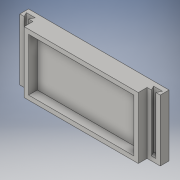
# Autodesk Inventor part: doveTailSide
Saved by Autodesk Inventor 2016 (Build 200138000, 138)
## iProperties
Created: 2015-11-04
Part Number: doveTailSide
Material: Generic
Document SubType Name: Modeling
Designer: rossmosier
Density: 1 g/cm^3
Appearance: Default
Author: rossmosier
Autodesk Inventor part; units mm, degrees
ref_plane "YZ Plane" through (0, 0, 0) normal (1, 0, 0) x (0, 1, 0)
ref_plane "XZ Plane" through (0, 0, 0) normal (0, 1, 0) x (-1, 0, 0)
ref_plane "XY Plane" through (0, 0, 0) normal (0, 0, 1) x (1, 0, 0)
sketch "Sketch2" plane through (0, 0, 0) normal (0, 0, 1) x (1, 0, 0)
  line L0 (0, 0) -> (203.2, 0)
  line L1 (203.2, 0) -> (203.2, 88.9)
  line L2 (203.2, 88.9) -> (0, 88.9)
  line L3 (0, 88.9) -> (0, 0)
  dimension "d6" = 203.2
  dimension "d7" = 88.9
  constraints: 8 end point, 2 parallel, 1 horizontal, 1 perpendicular
  measures "d6" distance of L2.end L1.end
  measures "d7" distance of L1.end L0.end
extrude "Extrusion2" add sketch "Sketch2" along normal blind 12.7
sketch "Sketch3" plane through (0, 0, 12.7) normal (0, 0, 1) x (1, 0, 0)
  line L0 (0, 0) -> (203.2, 0) projected
  line L1 (203.2, 0) -> (203.2, 88.9) projected
  line L2 (203.2, 88.9) -> (0, 88.9) projected
  line L3 (0, 88.9) -> (0, 0) projected
  line L4 (203.2, 88.9) -> (0, 88.9) construction
  line L5 (0, 0) -> (203.2, 0) construction
  line L6 (0, 88.9) -> (203.2, 0) construction
  line L7 (203.2, 0) -> (203.2, 88.9) construction
  line L8 (203.2, 88.9) -> (0, 0) construction
  line L9 (25.4, 6.35) -> (177.8, 6.35)
  line L10 (177.8, 6.35) -> (177.8, 82.55)
  line L11 (177.8, 82.55) -> (25.4, 82.55)
  line L12 (25.4, 82.55) -> (25.4, 6.35)
  line L13 (25.4, 6.35) -> (177.8, 82.55) construction
  line L14 (177.8, 6.35) -> (25.4, 82.55) construction
  line L15 (19.05, 88.9) -> (184.15, 88.9)
  line L16 (184.15, 88.9) -> (184.15, 0)
  line L17 (184.15, 0) -> (19.05, 0)
  line L18 (19.05, 0) -> (19.05, 88.9)
  point P0 (101.6, 44.45)
  dimension "d10" = 152.4
  dimension "d11" = 76.2
  dimension "d12" = 6.35
  constraints: 24 end point, 4 parallel, 3 midpoint, 2 perpendicular, 1 horizontal, 3 other
  measures "d10" distance of L11.end L10.end
  measures "d11" distance of L10.end L9.end
  measures "d12" distance between parallel lines of L11 L15
extrude "Extrusion3" add sketch "Sketch3" along normal blind 12.7 contours L18 L2 L16 L0
sketch "Sketch5" plane through (0, 88.9, 0) normal (0, 1, 0) x (1, 0, 0)
  line L0 (203.2, 0) -> (0, 0) projected
  line L1 (0, 0) -> (0, -12.7) projected
  line L2 (19.05, -12.7) -> (0, -12.7) projected
  line L3 (19.05, -12.7) -> (19.05, -25.4) projected
  line L4 (184.15, -25.4) -> (19.05, -25.4) projected
  line L5 (184.15, -12.7) -> (184.15, -25.4) projected
  line L6 (203.2, -12.7) -> (184.15, -12.7) projected
  line L7 (203.2, 0) -> (203.2, -12.7) projected
  line L8 (0, 0) -> (203.2, 0) construction
  line L9 (0, -12.7) -> (19.05, -12.7)
  line L10 (19.05, -12.7) -> (19.05, 0) construction
  line L11 (19.05, 0) -> (0, 0) construction
  line L12 (0, 0) -> (0, -12.7) construction
  line L13 (19.05, -12.7) -> (0, -12.7) construction
  line L14 (9.525, -12.7) -> (9.525, -6.3424) construction
  line L15 (9.525, -12.7) -> (12.7, -12.7) construction
  line L16 (9.525, -12.7) -> (6.35, -12.7)
  line L17 (9.525, -6.3424) -> (15.875, -6.3424)
  line L18 (9.525, -6.3424) -> (3.175, -6.3424)
  line L19 (3.175, -6.3424) -> (6.35, -12.7)
  line L20 (6.35, -12.7) -> (-12.7, -12.7)
  line L21 (193.6826, 0) -> (193.675, -12.7) construction
  line L22 (193.675, -12.7) -> (196.85, -12.7)
  line L23 (184.15, -12.7) -> (203.2, -12.7) projected
  line L24 (193.675, -12.7) -> (190.5, -12.7)
  line L25 (193.6788, -6.35) -> (187.3288, -6.35)
  line L26 (200.0288, -6.35) -> (196.85, -12.7)
  line L27 (187.3288, -6.35) -> (190.5, -12.7)
  line L28 (193.675, -12.7) -> (193.6788, -6.35) construction
  line L29 (9.525, -12.7) -> (9.525, -6.35) construction
  line L30 (15.875, -6.3424) -> (12.7, -12.7)
  line L31 (193.6788, -6.35) -> (200.0288, -6.35)
  line L32 (187.3288, -6.35) -> (200.0288, -6.35)
  line L33 (200.0288, -6.35) -> (196.85, -12.7)
  line L34 (196.85, -12.7) -> (190.5, -12.7)
  line L35 (187.3288, -6.35) -> (190.5, -12.7)
  line L36 (3.175, -6.3424) -> (6.35, -12.7)
  line L37 (6.35, -12.7) -> (12.7, -12.7)
  line L38 (12.7, -12.7) -> (15.875, -6.3424)
  line L39 (15.875, -6.3424) -> (3.175, -6.3424)
  dimension "d15" = 3.175
  dimension "d16" = 3.175
  dimension "d17" = 6.35
  dimension "d18" = 6.35
  dimension "d19" = 3.175
  dimension "d20" = 3.175
  dimension "d21" = 6.35
  dimension "d22" = 6.35
  dimension "d25" = 6.35
  dimension "d26" = 6.35
  constraints: 58 end point, 8 point on line, 6 collinear, 6 horizontal, 4 midpoint, 3 parallel, 1 perpendicular, 1 vertical
  measures "d15" distance of L14.start L15.end
  measures "d16" distance of L14.start L16.end
  measures "d17" distance of L14.end L17.end
  measures "d18" distance of L14.end L18.end
  measures "d19" distance of L21.end L22.end
  measures "d20" distance of L21.end L24.end
  measures "d21" distance of L25.start L25.end
  measures "d22" distance of L25.start L26.start
  measures "d25" distance of L21.end L28.end
  measures "d26" distance of L14.start L29.end
extrude "Extrusion5" cut sketch "Sketch5" against normal blind 82.55 contours L6 L27 L25 L31 L26 | L19 L18 L17 L30 L2
body "Solid2"
